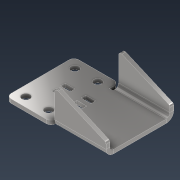
# Autodesk Inventor part: SP10V1 Estructura Freno
Saved by Autodesk Inventor 2021.2 (Build 252289000, 289)
## iProperties
Created: 2026-06-23
Part Number: SP10V1 Estructura Freno
Material: Generic
Document SubType Name: Sheet Metal
Designer: nelso
Density: 1 g/cm^3
Flat Pattern Width: 10.4006 cm
Flat Pattern Length: 8.4325 cm
Flat Pattern Area: 87.7032 cm^2
Sheet Metal Rule: Default_mm
Sheet Metal Width: 104.006 mm
Sheet Metal Length: 84.325 mm
Sheet Metal Area: 8770.320 mm^2
Appearance: Semi-Polished
Author: nelso
Autodesk Inventor part; units mm, degrees
ref_plane "YZ Plane" through (0, 0, 0) normal (1, 0, 0) x (0, 1, 0)
ref_plane "XZ Plane" through (0, 0, 0) normal (0, 1, 0) x (-1, 0, 0)
ref_plane "XY Plane" through (0, 0, 0) normal (0, 0, 1) x (1, 0, 0)
sketch "Sketch1" plane through (0, 0, 0) normal (0, 1, 0) x (-1, 0, 0)
  line L0 (-20, 28.6) -> (20, 28.6)
  line L1 (20, 28.6) -> (20, -28.6)
  line L2 (20, -28.6) -> (-20, -28.6)
  line L3 (-20, -28.6) -> (-20, 28.6)
  line L4 (-20, 28.6) -> (20, -28.6) construction
  line L5 (20, 28.6) -> (-20, -28.6) construction
  line L6 (20, 28.6) -> (20, 20.7)
  line L7 (20, 20.7) -> (11.3, 20.7)
  line L8 (-20, 28.6) -> (-18.4, 28.6)
  line L9 (-20, 20.7) -> (-20, 28.6)
  line L10 (27.1, -28.6) -> (18.4, -28.6)
  line L11 (27.1, -20.7) -> (27.1, -28.6)
  line L12 (-20, -28.6) -> (-25.5, -28.6)
  line L13 (-20, -20.7) -> (-20, -28.6)
  circle A0 centre (11.3, 20.7) radius 3.35
  circle A1 centre (-8, 20.7) radius 3.35
  circle A2 centre (-8, -20.7) radius 3.35
  line L14 (-20, 28.6) -> (-64.325, 28.6)
  line L15 (-64.325, 28.6) -> (-64.325, -28.6)
  line L16 (-64.325, -28.6) -> (-20, -28.6)
  line L17 (-20, -28.6) -> (-20, 28.6)
  line L18 (-64.325, -28.6) -> (-24.325, -28.6)
  line L19 (-64.325, 28.6) -> (-27.1, 28.6)
  line L20 (20, 0) -> (0.15, 0)
  line L21 (0.15, 6.0647) -> (0.15, 0)
  line L22 (0.15, 0) -> (-7.35, 0)
  line L23 (-7.35, 0) -> (-7.35, 6.0647)
  line L24 (-7.35, 0) -> (-17.35, 0)
  line L25 (-17.35, 0) -> (-17.35, 5.7069)
  line L26 (-17.35, 0) -> (-24.85, 0)
  line L27 (-24.85, 0) -> (-24.85, 5.7069)
  line L28 (-24.85, 0) -> (-41.05, 0)
  line L29 (-41.05, 0) -> (-41.05, 8.0124)
  line L30 (0, 0) -> (0, 1.4)
  line L31 (0, 0) -> (0, -1.279)
  circle A3 centre (11.3, -20.7) radius 3.35
  dimension "d0" = 40
  dimension "d1" = 57.2
  dimension "d2" = 7.9
  dimension "d3" = 8.7
  dimension "d11" = 6.7
  dimension "d12" = 6.7
  dimension "d15" = 57.2
  dimension "d73" = 19.85
  dimension "d74" = 7.5
  dimension "d75" = 10
  dimension "d76" = 7.5
  dimension "d77" = 16.2
  dimension "d78" = 1.4
  dimension "d99" = 7.9
  dimension "d100" = 7.9
  dimension "d107" = 8.7
  dimension "d108" = 7.9
  dimension "d109" = 6.7
  dimension "d110" = 6.7
  dimension "d111" = 12
  dimension "d112" = 12
  dimension "d113" = 44.325
  measures "d0" distance of L1.end L2.end
  measures "d1" distance of L0.end L1.end
  measures "d2" distance of L0.end L6.end
  measures "d3" distance of L6.end L7.end
  measures "d11" diameter of A1
  measures "d12" diameter of A2
  measures "d15" distance of L15.end L14.end
  measures "d73" distance of L20.start L20.end
  measures "d74" distance of L20.end L22.end
  measures "d75" distance of L22.end L24.end
  measures "d76" distance of L24.end L26.end
  measures "d77" distance of L26.end L28.end
  measures "d78" distance of L30.start L30.end
  measures "d99" distance from line of L0 A1.centre
  measures "d100" distance from line of L2 A2.centre
  measures "d107" distance from line of L1 A3.centre
  measures "d108" distance from line of L2 A3.centre
  measures "d109" diameter of A3
  measures "d110" diameter of A0
  measures "d111" distance from line of L3 A2.centre
  measures "d112" distance from line of L3 A1.centre
  measures "d113" distance between parallel lines of L3 L15
extrude "Plate1" add sketch "Sketch1" along normal blind 3.2
sketch "Sketch5" plane through (64.325, 0, 25.4) normal (0, 0, 1) x (1, 0, 0)
  line L0 (-43.325, 0) -> (0, 0)
  line L1 (0, 0) -> (0, 30)
  line L2 (0, 30) -> (-43.325, 30)
  line L3 (-43.325, 30) -> (-43.325, 0)
  constraints: 6 end point, 1 horizontal, 1 perpendicular, 1 vertical
edge flange "Flange3" height 30 angle 90 thickness 3.2 bend radius 3.2 thickness toward (0, 0, 1) relief straight relief width 3.2 relief depth 1.6 edges at (22.1625, 3.2, 28.6) wall of the first edge with corners at (21, 0, 25.4) (64.325, 0, 25.4) (64.325, 30, 25.4) (21, 30, 25.4)
bend "Bend3"
corner "Corner3"
sketch "Sketch6" plane through (-20, 0, -25.4) normal (0, 0, -1) x (-1, 0, 0)
  line L0 (-84.325, 0) -> (-41, 0)
  line L1 (-41, 0) -> (-41, 30)
  line L2 (-41, 30) -> (-84.325, 30)
  line L3 (-84.325, 30) -> (-84.325, 0)
  constraints: 8 end point
edge flange "Flange4" height 30 angle 90 thickness 3.2 bend radius 3.2 thickness toward (0, 0, -1) relief straight relief width 3.2 relief depth 1.6 edges at (22.1625, 3.2, -28.6) wall of the first edge with corners at (64.325, 0, -25.4) (21, 0, -25.4) (21, 30, -25.4) (64.325, 30, -25.4)
bend "Bend4"
corner "Corner4"
sketch "Sketch11" plane through (0, 3.2, 0) normal (0, 1, 0) x (1, 0, 0)
  line L0 (-4.61, 1.75) -> (-4.61, 4.95)
  line L1 (-4.61, 4.95) -> (-5.76, 4.95)
  line L2 (-5.76, 4.95) -> (-5.76, 1.75)
  line L3 (12.89, 1.75) -> (12.89, 4.95)
  line L4 (12.89, 4.95) -> (11.74, 4.95)
  line L5 (11.74, 4.95) -> (11.74, 1.75)
  line L6 (11.74, 1.75) -> (12.89, 1.75)
  line L7 (-4.61, -4.95) -> (-4.61, -1.75)
  line L8 (-4.61, -1.75) -> (2.89, -1.75)
  line L9 (2.89, -1.75) -> (2.89, -4.95)
  line L10 (2.89, -4.95) -> (-4.61, -4.95)
  line L11 (12.89, -4.95) -> (12.89, -1.75)
  line L12 (12.89, -1.75) -> (20.39, -1.75)
  line L13 (20.39, -1.75) -> (20.39, -4.95)
  line L14 (20.39, -4.95) -> (12.89, -4.95)
  line L15 (-4.61, 1.75) -> (3.69, 1.75)
  line L16 (3.69, 1.75) -> (3.69, 5.75)
  line L17 (3.69, 5.75) -> (-4.61, 5.75)
  line L18 (-4.61, 5.75) -> (-4.61, 1.75)
  line L19 (-4.61, -1.75) -> (3.69, -1.75)
  line L20 (3.69, -1.75) -> (3.69, -5.75)
  line L21 (3.69, -5.75) -> (-4.61, -5.75)
  line L22 (-4.61, -5.75) -> (-4.61, -1.75)
  line L23 (12.89, -1.75) -> (21.19, -1.75)
  line L24 (21.19, -1.75) -> (21.19, -5.75)
  line L25 (21.19, -5.75) -> (12.89, -5.75)
  line L26 (12.89, -5.75) -> (12.89, -1.75)
  line L27 (12.89, 1.75) -> (21.19, 1.75)
  line L28 (21.19, 1.75) -> (21.19, 5.75)
  line L29 (21.19, 5.75) -> (12.89, 5.75)
  line L30 (12.89, 5.75) -> (12.89, 1.75)
  line L31 (-20, -28.6) -> (-20, 28.6) projected
  point P0 (0, 0)
  dimension "d89" = 8.3
  dimension "d90" = 4
  dimension "d91" = 8.3
  dimension "d92" = 4
  dimension "d93" = 8.3
  dimension "d94" = 4
  dimension "d95" = 8.3
  dimension "d96" = 4
  dimension "d114" = 15.39
  dimension "d115" = 9.2
  dimension "d116" = 9.2
  dimension "d117" = 3.5
  dimension "d118" = 3.5
  dimension "d120" = 15.39
  constraints: 62 end point, 8 parallel, 4 horizontal, 4 perpendicular
  measures "d89" distance of L17.end L16.end
  measures "d90" distance of L16.end L15.end
  measures "d91" distance of L20.end L21.end
  measures "d92" distance of L19.end L20.end
  measures "d93" distance of L24.end L25.end
  measures "d94" distance of L23.end L24.end
  measures "d95" distance of L29.end L28.end
  measures "d96" distance of L28.end L27.end
  measures "d114" distance between parallel lines of L7 L31
  measures "d115" distance between parallel lines of L20 L11
  measures "d116" distance between parallel lines of L16 L3
  measures "d117" distance between parallel lines of L6 L12
  measures "d118" distance between parallel lines of L15 L8
  measures "d120" distance between parallel lines of L31 L0
extrude "Cut3" cut sketch "Sketch11" against normal blind 3.2 contours L0 L18 L17 L16 L15 | L3 L30 L29 L28 L27 | L7 L8 L9 L10 | L10 L9 L19 L20 L21 L22 | L11 L12 L13 L14 | L14 L13 L23 L24 L25 L26
fillet "Corner Round1" radius 4 4 edges at (-20, 1.6, -28.6) (-20, 1.6, 28.6) (17.8, 1.6, 28.6) (17.8, 1.6, -28.6)
sketch "Sketch12" plane through (64.325, 30, -28.6) normal (0, 0, -1) x (-1, 0, 0)
  line L0 (0, -23.6) -> (43.325, -23.6) projected
  line L1 (0, -23.6) -> (0, -18.6)
  line L2 (0, 0) -> (0, -23.6) projected
  line L3 (43.325, 0) -> (0, 0) projected
  line L4 (0, -18.6) -> (43.325, 0)
  line L5 (43.325, 0) -> (43.325, -18.6)
  line L6 (43.325, -23.6) -> (43.325, 0) projected
  line L7 (0, -18.6) -> (43.325, -18.6)
  point P0 (64.325, -30)
  dimension "d102" = 5
  constraints: 8 end point, 2 point on line, 1 perpendicular
  measures "d102" distance of L0.start L1.end
extrude "Cut4" cut sketch "Sketch12" against normal up to surface (57.2 mm away) contours L2 L3 L4
fillet "Corner Round2" radius 2 4 edges at (21, 30, 27) (21, 30, -27) (64.325, 11.4, 27) (64.325, 11.4, -27)
equation "\"d99\" = d2"
equation "\"d100\" = d99"
equation "\"d107\" = d3"
equation "\"d108\" = d2"
equation "\"d109\" = d10"
equation "\"d97\" = Thickness"
equation "\"d103\" = Thickness"
equation "\"d22\" = Thickness"
equation "\"d49\" = BendReliefWidth"
equation "\"d50\" = BendReliefDepth"
equation "\"d51\" = MinimumRemnant"
equation "\"d52\" = TransitionRadius"
equation "\"d57\" = BendRadius"
equation "\"d58\" = CornerReliefSize"
equation "\"d59\" = GapSize"
equation "\"d60\" = JacobiRadiusSize"
equation "\"d61\" = BendReliefWidth"
equation "\"d62\" = BendReliefDepth"
equation "\"d63\" = MinimumRemnant"
equation "\"d64\" = TransitionRadius"
equation "\"d69\" = BendRadius"
equation "\"d70\" = CornerReliefSize"
equation "\"d71\" = GapSize"
equation "\"d72\" = JacobiRadiusSize"
equation "\"d89\" = d91"
equation "\"d90\" = d92"
equation "\"d93\" = d91"
equation "\"d94\" = d92"
equation "\"d95\" = d91"
equation "\"d96\" = d92"
equation "\"d116\" = d115"
equation "\"d117\" = d118"
equation "\"d120\" = d114"
equation "\"BendRadius\" = Thickness"
equation "\"BendReliefWidth\" = Thickness"
equation "\"BendReliefDepth\" = 0.5 * Thickness"
equation "\"CornerReliefSize\" = 4 * Thickness"
equation "\"MinimumRemnant\" = 2 * Thickness"
equation "\"TransitionRadius\" = BendRadius"
equation "\"JacobiRadiusSize\" = BendRadius"
equation "\"GapSize\" = Thickness"
equation "\"d10\" = 6.7"
equation "\"Thickness\" = 3.2"
body "Solid1"
